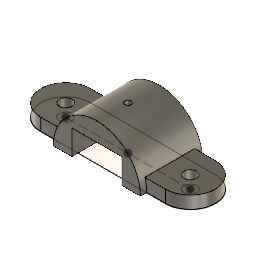
ch7example v2 (Autodesk Fusion 360 design; units mm, degrees)
Autodesk Fusion 360 part; units mm, degrees
note: some values were not read from the file. Chosen so that the rebuilt part matches the saved one: a direction.
sketch "Sketch1" plane through (0, 0, 0) normal (0, 0, 1) x (1, 0, 0) in component "u-Bracket"
  line L0 (-63.5, -25.4) -> (63.5, -25.4)
  arc A0 (63.5, -25.4) -> (63.5, 25.4) centre (63.5, 0) ccw
  line L1 (63.5, 25.4) -> (-63.5, 25.4)
  arc A1 (-63.5, 25.4) -> (-63.5, -25.4) centre (-63.5, 0) ccw
  line L2 (-63.5, 0) -> (63.5, 0) construction
  circle A2 centre (63.5, 0) radius 6.35
  circle A3 centre (-63.5, 0) radius 6.35
  dimension "d1" = 127
  dimension "d2" = 12.7
  dimension "d3" = 12.7
  dimension "d4" = 25.4
  dimension "d5" = 63.5
  measures "d2" diameter of A2
  measures "d3" diameter of A3
  measures "d4" radius of A0
extrude "Extrude2" add sketch "Sketch1" along normal blind 12.7 makes body 1 in component "u-Bracket"
extrude "Extrude1" add sketch "Sketch1" along normal blind 12.7 separate body makes body 2 in component "u-Bracket"
sketch "Sketch2" plane through (0, 0, 0) normal (0, 1, 0) x (1, 0, 0) in component "u-Bracket"
  circle A0 centre (0, 0) radius 44.45
  line L0 (-44.45, 0) -> (44.45, 0)
  dimension "d10" = 88.9
  measures "d10" diameter of A0
extrude "Extrude3" add sketch "Sketch2" along normal mid plane 63.5 contours A0 L0 picked at (-7.4083, -12.8316) bodies 1 2 in component "u-Bracket"
sketch "Sketch3" plane through (0, -31.75, 0) normal (0, -1, 0) x (1, 0, 0) in component "u-Bracket"
  arc A0 (44.45, 0) -> (-44.45, 0) centre (0, 0) ccw
  line L0 (-44.45, 0) -> (44.45, 0)
  line L1 (-25.4, 0) -> (25.4, 0)
  line L2 (25.4, 0) -> (25.4, 25.4)
  line L3 (25.4, 25.4) -> (-25.4, 25.4)
  line L4 (-25.4, 25.4) -> (-25.4, 0)
  line L5 (-63.5, 0) -> (63.5, 0)
  dimension "d13" = 50.8
  dimension "d14" = 25.4
extrude "Extrude4" cut sketch "Sketch3" against normal through all contours L0 L1 L2 L3 L4 L5 bodies 1 in component "u-Bracket"
sketch "Sketch4" plane through (0, 0, 25.4) normal (0, 0, -1) x (1, 0, 0) in component "u-Bracket"
  line L0 (-25.4, -31.75) -> (25.4, -31.75)
  line L1 (25.4, -31.75) -> (25.4, 31.75)
  line L2 (25.4, 31.75) -> (-25.4, 31.75)
  line L3 (-25.4, 31.75) -> (-25.4, -31.75)
  circle A0 centre (0, 0) radius 3.175
  dimension "d16" = 6.35
  measures "d16" diameter of A0
extrude "Extrude5" cut sketch "Sketch4" against normal through all contours A0 bodies 1 in component "u-Bracket"
component "u-Bracket" placed x (1, 0, 0) y (0, 1, 0) z (0, 0, 1) at (0, 0, 0)
equation "d5 = d1 / 2"
